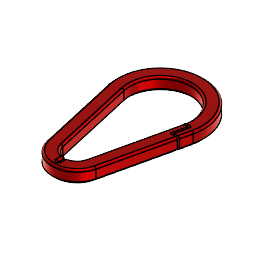
Carabiner (Autodesk Fusion 360 design; units mm, degrees)
part number: 2026-06-10-22-35-48-990
Autodesk Fusion 360 part; units mm, degrees
sketch "Sketch1" plane through (0, 0, 0) normal (0, 0, 1) x (1, 0, 0)
  line L0 (-19.4999, 50.5556) -> (-9.75, 7.7778)
  line L1 (19.4999, 50.5556) -> (9.75, 7.7778)
  arc A0 (19.4999, 50.5556) -> (-19.4999, 50.5556) centre (0, 55) ccw
  arc A1 (-9.75, 7.7778) -> (9.75, 7.7778) centre (0, 10) ccw
  dimension "d1" = 55
  dimension "d2" = 40
  dimension "d3" = 20
  constraint vertical A0.centre A1.centre
  constraint vertical origin A1.centre
  constraint coincident origin A1
  constraint tangent L0 A1
  constraint tangent L0 A0
  constraint tangent L1 A0
  constraint tangent L1 A1
  measures "d1" distance of origin A0.centre
  measures "d2" diameter of A0
  measures "d3" diameter of A1
sketch "Sketch4" plane through (0, 0, 0) normal (1, 0, 0) x (0, 1, 0)
  line L0 (3.5, 3.5) -> (-3.5, 3.5)
  line L1 (-3.5, 3.5) -> (-3.5, -3.5)
  line L2 (-3.5, -3.5) -> (3.5, -3.5)
  line L3 (3.5, -3.5) -> (3.5, 3.5)
  line L4 (3.5, 3.5) -> (-3.5, -3.5) construction
  line L5 (-3.5, 3.5) -> (3.5, -3.5) construction
  dimension "d4" = 7
  dimension "d5" = 7
  constraint horizontal L0
  constraint perpendicular L0 L1
  constraint parallel L0 L2
  constraint parallel L1 L3
  constraint coincident L4 origin
  constraint coincident L5 origin
  measures "d4" distance of L0.start L0.end
  measures "d5" distance of L0.end L1.end
sweep "Sweep1" add profiles "Sketch4" path "Sketch1" along A1 L0 A0 L1 section 1
chamfer "Chamfer1" distance 1.5 angle 45 4 faces at (-14.1374, 21.7778, -3.5) (-2.3205, -0.8922, -3.5) (11.8625, 22.2963, -3.5) (-7.3276, 74.799, -3.5)
sketch "Sketch5" plane through (0, 0, 3.5) normal (0, 0, 1) x (-1, 0, 0)
  line L0 (22.9124, -49.7778) -> (13.1624, -7)
  arc A0 (13.1624, -7) -> (-13.1624, -7) centre (0, -10) ccw
  line L1 (-13.1624, -7) -> (-22.9124, -49.7778)
  arc A1 (-22.9124, -49.7778) -> (22.9124, -49.7778) centre (0, -55) ccw
  arc A2 (-16.0874, -51.3333) -> (16.0874, -51.3333) centre (0, -55) ccw
  line L2 (-16.0874, -51.3333) -> (-6.3375, -8.5556)
  arc A3 (6.3375, -8.5556) -> (-6.3375, -8.5556) centre (0, -10) ccw
  line L3 (6.3375, -8.5556) -> (16.0874, -51.3333)
  line L4 (-0.5, 0) -> (-0.5, -3.5)
  arc A4 (-0.5, -3.5) -> (0.5, -3.5) centre (0, -3.5) ccw
  line L5 (0.5, -3.5) -> (0.5, 0)
  arc A5 (0.5, 0) -> (-0.5, 0) centre (0, 0) ccw
  line L6 (0, 0) -> (0, -3.5) construction
  dimension "d13" = 1
  constraint tangent L4 A4
  constraint tangent A4 L5
  constraint parallel L4 L5
  constraint tangent L5 A5
  constraint tangent L4 A5
  constraint midpoint A3 A4.centre
  constraint vertical L6
  constraint coincident A5.centre L6.start
  measures "d13" diameter of A4
extrude "Extrude1" cut sketch "Sketch5" against normal blind 7 contours A3 L4 A4 L5 A5
sketch "Sketch8" plane through (0, 0, 3.5) normal (0, 0, 1) x (-1, 0, 0)
  arc A0 (-0.5, -3.5) -> (-0.4996, -3.5192) centre (0, -3.5) ccw
  line L0 (-0.5, -3.5) -> (-0.5, 0)
  arc A1 (0.5, 0) -> (-0.5, 0) centre (0, 0) ccw
  line L1 (0.5, 0) -> (0.5, -3.5)
  arc A2 (0.4996, -3.5192) -> (0.5, -3.5) centre (0, -3.5) ccw
  arc A3 (6.3375, -8.5556) -> (0.4996, -3.5192) centre (0, -10) ccw
  line L2 (6.3375, -8.5556) -> (16.0874, -51.3333)
  arc A4 (-16.0874, -51.3333) -> (16.0874, -51.3333) centre (0, -55) ccw
  line L3 (-16.0874, -51.3333) -> (-6.3375, -8.5556)
  arc A5 (-0.4996, -3.5192) -> (-6.3375, -8.5556) centre (0, -10) ccw
  line L4 (22.9124, -49.7778) -> (13.1624, -7)
  arc A6 (13.1624, -7) -> (-13.1624, -7) centre (0, -10) ccw
  line L5 (-13.1624, -7) -> (-22.9124, -49.7778)
  arc A7 (-22.9124, -49.7778) -> (22.9124, -49.7778) centre (0, -55) ccw
  arc A8 (-16.0874, -51.3333) -> (16.0874, -51.3333) centre (0, -55) ccw
  line L6 (-16.0874, -50.8333) -> (-19.6772, -50.8333)
  arc A9 (-19.6772, -50.8333) -> (-19.6772, -51.8333) centre (-19.6772, -51.3333) ccw
  line L7 (-19.6772, -51.8333) -> (-16.0874, -51.8333)
  arc A10 (-16.0874, -51.8333) -> (-16.0874, -50.8333) centre (-16.0874, -51.3333) ccw
  line L8 (-16.0874, -51.3333) -> (-19.6772, -51.3333) construction
  line L9 (-19.1897, -51.4444) -> (-17.3663, -43.4444)
  arc A11 (-17.3663, -43.4444) -> (-18.3413, -43.2222) centre (-17.8538, -43.3333) ccw
  line L10 (-18.3413, -43.2222) -> (-20.1647, -51.2222)
  arc A12 (-20.1647, -51.2222) -> (-19.1897, -51.4444) centre (-19.6772, -51.3333) ccw
  line L11 (-19.6772, -51.3333) -> (-17.8538, -43.3333) construction
  line L12 (-21.4436, -43.8333) -> (-17.8538, -43.8333)
  arc A13 (-17.8538, -43.8333) -> (-17.8538, -42.8333) centre (-17.8538, -43.3333) ccw
  line L13 (-17.8538, -42.8333) -> (-21.4436, -42.8333)
  arc A14 (-21.4436, -42.8333) -> (-21.4436, -43.8333) centre (-21.4436, -43.3333) ccw
  line L14 (-21.4436, -43.3333) -> (-17.8538, -43.3333) construction
  dimension "d16" = 0.5
  dimension "d17" = 8
  constraint tangent L6 A9
  constraint tangent A9 L7
  constraint parallel L6 L7
  constraint tangent L7 A10
  constraint tangent L6 A10
  constraint horizontal L8
  constraint coincident A4.start L3.start
  constraint tangent L9 A11
  constraint tangent A11 L10
  constraint parallel L9 L10
  constraint tangent L10 A12
  constraint tangent L9 A12
  constraint coincident A9.centre L8.end
  constraint tangent L12 A13
  constraint tangent A13 L13
  constraint parallel L12 L13
  constraint tangent L13 A14
  constraint tangent L12 A14
  constraint coincident A11.centre L11.end
  constraint horizontal L14
  constraint coincident L5 A14.centre
  constraint equal L8 L14
  constraint equal A11 A13
  constraint equal A10 A12
  constraint parallel L3 L11
  measures "d16" radius of A14
  measures "d17" vertical distance of A4.start A11.centre
fillet "Fillet1" radius 1 1 faces at (-17.3874, 36.037, 3.5)
extrude "Extrude2" cut sketch "Sketch8" against normal blind 7 contours A4 L3 A8 L7 A10 | A4 L3 A8 L6 L7 A10 L9 A12 | L6 A9 L9 A12 | L6 A9 L9 L10 L12 A13 | A11 L10 L12 A13 | L5 A11 L10 L12 L13 A14 | L5 L13 A14
